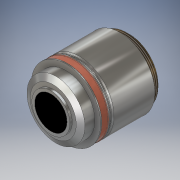
# Autodesk Inventor part: ZEISS EC Epiplan-Neofluar (422320-9900-000)
Saved by Autodesk Inventor 2017 (Build 210142000, 142)
## iProperties
Part Number: ZEISS EC Epiplan-Neofluar (422320-9900-000)
Material: Generisch
Document SubType Name: Modeling
Designer: ExCISS
Density: 1 g/cm^3
Appearance: Chrom - poliert
Author: ExCISS
Autodesk Inventor part; units mm, degrees
ref_plane "YZ Plane" through (0, 0, 0) normal (1, 0, 0) x (0, 1, 0)
ref_plane "XZ Plane" through (0, 0, 0) normal (0, 1, 0) x (-1, 0, 0)
ref_plane "XY Plane" through (0, 0, 0) normal (0, 0, 1) x (1, 0, 0)
sketch "Skizze1" plane through (0, 0, 0) normal (0, 0, 1) x (1, 0, 0)
  line L0 (0, 146.3203) -> (0, -146.3203) construction
  line L1 (7, -16.9) -> (7, 16.9)
  line L2 (7, 16.9) -> (12.5, 16.9)
  line L3 (12.5, 16.9) -> (12.5, 15.9)
  line L4 (12.5, 15.9) -> (13.5, 15.9)
  line L5 (13.5, 15.9) -> (13.5, 14)
  line L6 (13.5, 14) -> (12.5, 14)
  line L7 (12.5, 14) -> (12.5, 13)
  line L8 (12.5, 13) -> (15, 13)
  line L9 (15, 13) -> (15, -4.65)
  line L10 (15, -4.65) -> (14.5, -5.15)
  line L11 (14.5, -5.15) -> (14.5, -5.65)
  line L12 (15, -6.4) -> (15, -6.9)
  line L13 (15, -6.9) -> (14.8, -7.1)
  line L14 (14.8, -7.1) -> (14.8, -9.7)
  line L15 (14.8, -9.7) -> (15, -9.9)
  line L16 (15, -9.9) -> (15, -10.4)
  line L17 (15, -10.4) -> (12.5, -10.4)
  line L18 (12.5, -10.4) -> (12.5, -14.7109)
  line L19 (12.5, -14.7109) -> (9.95, -15.9)
  line L20 (9.95, -15.9) -> (8.225, -15.9)
  line L21 (8.225, -15.9) -> (8.225, -16.9)
  line L22 (8.225, -16.9) -> (7, -16.9)
  line L23 (15, -6.4) -> (14.567, -5.65)
  line L24 (14.567, -5.65) -> (14.5, -5.65)
  line L25 (0, 0) -> (7, 0) construction
  dimension "d0" = 15
  dimension "d1" = 29.9
  dimension "d2" = 3.9
  dimension "d3" = 25
  dimension "d7" = 28.9
  dimension "d8" = 23.4
  dimension "d11" = 1
  dimension "d12" = 1
  dimension "d13" = 14.8
  dimension "d14" = 2.6
  dimension "d15" = 14.5
  dimension "d16" = 1.75
  dimension "d17" = 0.5
  dimension "d18" = 0.5
  dimension "d19" = 8.225
  dimension "d20" = 9.95
  dimension "d21" = 12.5
  dimension "d22" = 13.5
  dimension "d23" = 12.5
  dimension "d24" = 45
  dimension "d25" = 30
  dimension "d26" = 45
  dimension "d27" = 0.75
  dimension "d28" = 7
  constraints: 52 end point, 13 perpendicular, 5 point on line, 3 vertical, 2 horizontal, 2 midpoint, 2 parallel, 1 coincident
  measures "d0" distance between parallel lines of L9 L0
  measures "d1" distance between parallel lines of L22 L8
  measures "d2" distance between parallel lines of L8 L2
  measures "d3" angle of L19 L20
  measures "d7" distance between parallel lines of L20 L8
  measures "d8" distance between parallel lines of L8 L17
  measures "d11" distance between parallel lines of L2 L4
  measures "d12" distance between parallel lines of L8 L6
  measures "d13" distance between parallel lines of L0 L14
  measures "d14" distance of L14.end L13.end
  measures "d15" distance between parallel lines of L0 L11
  measures "d16" distance of L12.start L9.end
  measures "d17" vertical distance of L15.end L17.end
  measures "d18" distance of L12.start L12.end
  measures "d19" distance from line of L0 L21.end
  measures "d20" distance from line of L0 L19.end
  measures "d21" distance from line of L0 L17.end
  measures "d22" distance between parallel lines of L0 L5
  measures "d23" distance between parallel lines of L0 L3
  measures "d24" angle of L11 L10
  measures "d25" angle of L23 L12
  measures "d26" angle of L16 L15
  measures "d27" distance from line of L24 L12.start
  measures "d28" distance between parallel lines of L1 L0
revolve "Umdrehung1" add sketch "Skizze1" angle 360 about axis through (0, 146.3203, 0) along (0, -1, 0)
thread "Gewinde1" size "M27x0.75" class "6g" standard "ANSI Metric M Profile" full length
ref_plane "image plane" through (0, -32, 0) normal (0, 1, 0) x (1, 0, 0)
